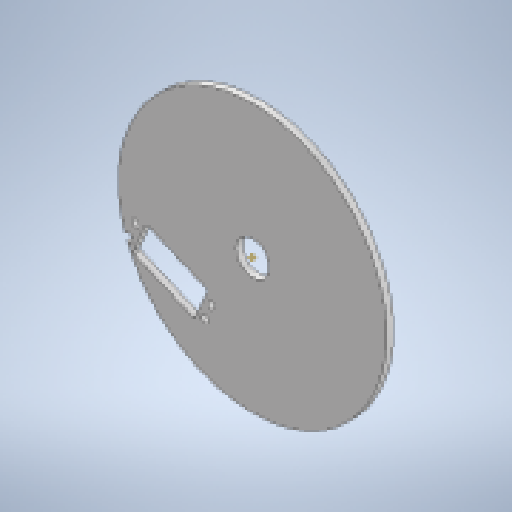
# Autodesk Inventor part: нижний эллипс головы
Saved by Autodesk Inventor 2023 (Build 270158000, 158)
## iProperties
Created: 2024-11-21
Part Number: нижний эллипс головы
Material: Типовые
Document SubType Name: Modeling
Designer: DELL
Density: 1 g/cm^3
Appearance: По умолчанию
Author: DELL
Autodesk Inventor part; units mm, degrees
ref_plane "YZ Plane" through (0, 0, 0) normal (1, 0, 0) x (0, 1, 0)
ref_plane "XZ Plane" through (0, 0, 0) normal (0, 1, 0) x (-1, 0, 0)
ref_plane "XY Plane" through (0, 0, 0) normal (0, 0, 1) x (1, 0, 0)
sketch "Эскиз1" plane through (0, 0, 0) normal (0, 0, 1) x (1, 0, 0)
  circle A0 centre (0, 0) radius 80
  line L0 (-73.0458, -9.1013) -> (-55.9791, -43.6261)
  line L1 (-55.8883, 0.3213) -> (-72.6635, -7.9712)
  circle A1 centre (-72.0801, -8.7984) radius 1
  circle A2 centre (-55.1518, -43.0425) radius 1.0002
  line L2 (-54.7582, -0.0611) -> (-37.6914, -34.586)
  circle A3 centre (-55.5854, -0.6446) radius 1.0001
  line L3 (-54.849, -44.0085) -> (-38.0739, -35.716)
  circle A4 centre (-38.6572, -34.8889) radius 1
  circle A5 centre (-48.8609, -46.2915) radius 2.2502
  circle A6 centre (-39.8964, -41.8599) radius 2.25
  circle A7 centre (-61.8764, 2.6041) radius 2.25
  circle A8 centre (-70.8409, -1.8274) radius 2.25
  point P0 (-58.3538, 3.8585)
  point P1 (-37.7608, -34.4457)
  point P2 (-38.2141, -35.7853)
  point P3 (-54.7086, -43.9391)
  point P4 (-56.0485, -43.4857)
  point P5 (-72.9765, -9.2415)
  point P6 (-72.5232, -7.9019)
  point P7 (-56.0286, 0.2519)
  point P8 (-54.6889, -0.2014)
  dimension "d2" = 160
  constraints: 9 centre point, 8 end point, 8 tangent, 1 coincident
  measures "d2" diameter of A0
extrude "Выдавливание1" add sketch "Эскиз1" against normal blind 4
sketch "Эскиз2" plane through (0, 0, 0) normal (0, 0, 1) x (1, 0, 0)
  circle A0 centre (0, 0) radius 80
  circle A1 centre (0, 0) radius 10
  dimension "d4" = 20
  constraints: 2 centre point
  measures "d4" diameter of A1
extrude "Выдавливание2" cut sketch "Эскиз2" against normal blind 10 contours A1
